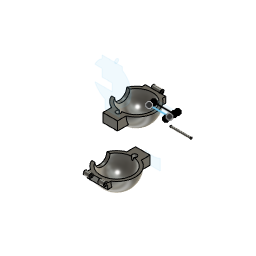
문고리 v1 (Autodesk Fusion 360 design; units mm, degrees)
Autodesk Fusion 360 part; units mm, degrees
sphere "구 기본체1" add diameter 65 placed x (1, 0, 0) y (0, 1, 0) z (0, 0, 1) at (0, 0, 0) makes body 1
split "분할1" by plane through (0, 0, 0) normal (0, 1, 0) bodies 1 makes body 2 at (30.8124, 7.6824, -6.9156)
move_body "이동1" bodies 2 to x (1, 0, 0) y (0, 1, 0) z (0, 0, 1) at (0, 40, 0)
move_body "이동2" bodies 2 to x (1, 0, 0) y (0, 1, 0) z (0, 0, 1) at (0, 80, 0)
sketch "스케치2" plane through (0, 120, 0) normal (0, -1, 0) x (1, 0, 0)
move_body "이동3" bodies 1 to x (1, 0, 0) y (0, 1, 0) z (0, 0, 1) at (190, 0, 0)
sketch "스케치3" plane through (0, 120, 0) normal (0, -1, 0) x (1, 0, 0)
  arc A0 (27.5, 0) -> (-27.5, 0) centre (0, 0) ccw
  line L0 (-27.5, 0) -> (27.5, 0)
  dimension "d2" = 27.5
  constraint coincident A0.centre origin
  constraint horizontal L0
  measures "d2" radius of A0
revolve "회전1" cut sketch "스케치3" angle 360 about axis through (-27.5, 120, 0) along (1, 0, 0) bodies 2
delete_body "본체 제거1" bodies 1
copy_body "CopyPasteBodies1" bodies 2 makes body 3
move_body "이동4" bodies 3 to x (1, 0, 0) y (0, 1, 0) z (0, 0, 1) at (130, 0, 0)
delete_body "본체 제거2" bodies 2
delete_body "본체 제거3" bodies 3
sphere "구 기본체2" add diameter 65 placed x (1, 0, 0) y (0, 1, 0) z (0, 0, 1) at (0, 0, 0) separate body makes body 4
sketch "스케치5" plane through (0, 0, 0) normal (0, 0, 1) x (1, 0, 0)
sketch "스케치6" plane through (0, 0, 0) normal (0, 0, 1) x (1, 0, 0)
  line L0 (-12.5, 0) -> (-12.5, 15)
  line L1 (-12.5, 15) -> (-12.5, -15)
  line L2 (-12.5, -15) -> (12.5, -15)
  line L3 (12.5, -15) -> (12.5, 15)
  line L4 (12.5, 15) -> (-12.5, 15)
  dimension "d7" = 12.5
  dimension "d9" = 15
  dimension "d10" = 30
  dimension "d11" = 25
  constraint perpendicular L1 L2
  constraint perpendicular L0 L4
  measures "d7" distance of origin L0.start
  measures "d9" distance of L0.start L0.end
  measures "d10" distance of L0.end L1.end
  measures "d11" distance of L1.end L2.end
extrude "돌출1" add sketch "스케치6" against normal blind 40 bodies 4
sketch "스케치7" plane through (0, 0, 0) normal (1, 0, 0) x (0, 1, 0)
  circle A0 centre (0, 0) radius 13
  dimension "d14" = 26
  constraint coincident A0.centre origin
  measures "d14" diameter of A0
extrude "돌출2" cut sketch "스케치7" against normal blind 32.5 bodies 4
extrude "돌출3" add 1 faces at (-4.1667, -5, -40) along direction (0, 0, -1) blind 10 on bodies 4 bodies 4
extrude "돌출4" cut 1 faces at (-4.1667, -5, -50) along direction (0, 0, 1) blind 5 on bodies 4 bodies 4
sketch "스케치8" plane through (0, -15, 0) normal (0, -1, 0) x (1, 0, 0)
  line L0 (-12.5, -45) -> (12.5, -45)
  line L1 (12.5, -45) -> (12.5, -25.9808)
  arc A0 (-12.5, -25.9808) -> (12.5, -25.9808) centre (0, 0) ccw
  line L2 (-12.5, -25.9808) -> (-12.5, -45)
sketch "스케치9" plane through (0, -15, 0) normal (0, -1, 0) x (1, 0, 0)
  circle A0 centre (0, -31) radius 4
  dimension "d21" = 8
  measures "d21" diameter of A0
extrude "돌출5" cut sketch "스케치9" along normal blind -65 and the other way blind -110 bodies 4
sketch "스케치10" plane through (0, 0, 0) normal (0, 0, 1) x (1, 0, 0)
  line L0 (17.5, 10) -> (-17.5, 10)
  line L1 (-17.5, 10) -> (-17.5, -10)
  line L2 (-17.5, -10) -> (17.5, -10)
  line L3 (17.5, -10) -> (17.5, 10)
  line L4 (17.5, 10) -> (-17.5, -10) construction
  line L5 (-17.5, 10) -> (17.5, -10) construction
  dimension "d26" = 35
  dimension "d27" = 20
  constraint horizontal L0
  constraint perpendicular L0 L1
  constraint parallel L0 L2
  constraint parallel L1 L3
  constraint coincident L4 origin
  constraint coincident L5 origin
  measures "d26" distance of L1.end L2.end
  measures "d27" distance of L0.end L1.end
extrude "돌출6" add sketch "스케치10" along normal blind 33 bodies 4
sketch "스케치11" plane through (0, 0, 33) normal (0, 0, 1) x (-1, 0, 0)
  line L0 (-17.5, 10) -> (-17.5, -10)
  line L1 (-17.5, -10) -> (17.5, -10)
  line L2 (17.5, -10) -> (17.5, 10)
  line L3 (17.5, 10) -> (-17.5, 10)
  line L4 (-17.5, 10) -> (-17.5, 4)
  line L5 (17.5, 4) -> (-17.5, 4)
  line L6 (-17.5, -10) -> (-17.5, -4)
  line L7 (-17.5, -4) -> (17.5, -4)
  dimension "d30" = 6
  constraint coincident L0.start L3.end
  constraint coincident L0 L4.end
  constraint perpendicular L3 L4
  constraint coincident L2 L5.start
  constraint perpendicular L4 L5
  constraint coincident L0.end L1.start
  constraint coincident L0 L6.end
  constraint coincident L2 L7.end
  constraint perpendicular L2 L7
  measures "d30" distance of L0.end L6.end
sketch "스케치12" plane through (17.5, 0, 0) normal (1, 0, 0) x (0, 1, 0)
  arc A0 (10, 25.4951) -> (-10, 25.4951) centre (0, 0) ccw
  line L0 (10, 25.4951) -> (10, 33)
  line L1 (10, 33) -> (-10, 33)
  line L2 (-10, 33) -> (-10, 25.4951)
  circle A1 centre (0, 36.5) radius 3.5
split "분할2" by plane through (0, 0, 0) normal (0, 1, 0) bodies 4 makes body 5 at (28.1333, 16.2428, -0.9692)
move_body "이동5" bodies 5 to x (1, 0, 0) y (0, 1, 0) z (0, 0, 1) at (-115, 30, 0)
sketch "스케치13" plane through (0, 30, 0) normal (0, -1, 0) x (1, 0, 0)
  line L0 (-127.5, -45) -> (-102.5, -45)
  line L1 (-102.5, -45) -> (-102.5, -30)
  arc A0 (-102.5, -30) -> (-97.5, 27.3861) centre (-115, 0) ccw
  line L2 (-97.5, 27.3861) -> (-97.5, 33)
  line L3 (-97.5, 33) -> (-132.5, 33)
  line L4 (-132.5, 33) -> (-132.5, 27.3861)
  arc A1 (-132.5, 27.3861) -> (-144.7867, 13) centre (-115, 0) ccw
  line L5 (-144.7867, 13) -> (-132.5, 13)
  line L6 (-132.5, 13) -> (-132.5, 0)
  line L7 (-132.5, 0) -> (-115, 0)
  line L8 (-115, 0) -> (-115, -13)
  line L9 (-115, -13) -> (-144.7867, -13)
  arc A2 (-144.7867, -13) -> (-127.5, -30) centre (-115, 0) ccw
  line L10 (-127.5, -30) -> (-127.5, -45)
  circle A3 centre (-115, -31) radius 4
sketch "스케치14" plane through (0, 30, 0) normal (0, -1, 0) x (1, 0, 0)
  arc A0 (-87.5, 0) -> (-142.5, 0) centre (-115, 0) ccw
  line L0 (-142.5, 0) -> (-87.5, 0)
  dimension "d31" = 27.5
  constraint horizontal L0
  measures "d31" radius of A0
sketch "스케치15" plane through (0, 30, 0) normal (0, -1, 0) x (1, 0, 0)
sketch "스케치16" plane through (0, 30, 0) normal (0, -1, 0) x (1, 0, 0)
revolve "회전2" cut sketch "스케치14" angle 360 about axis through (-142.5, 30, 0) along (1, 0, 0) bodies 5
sketch "스케치17" plane through (0, 0, 0) normal (0, 1, 0) x (-1, 0, 0)
  circle A0 centre (0, -31) radius 4
  line L0 (-12.5, -45) -> (12.5, -45)
  line L1 (12.5, -45) -> (12.5, -30)
  arc A1 (12.5, -30) -> (29.7867, -13) centre (0, 0) ccw
  line L2 (29.7867, -13) -> (0, -13)
  line L3 (0, -13) -> (0, 0)
  line L4 (0, 0) -> (17.5, 0)
  line L5 (17.5, 0) -> (17.5, 13)
  line L6 (17.5, 13) -> (29.7867, 13)
  arc A2 (29.7867, 13) -> (17.5, 27.3861) centre (0, 0) ccw
  line L7 (17.5, 27.3861) -> (17.5, 33)
  line L8 (17.5, 33) -> (-17.5, 33)
  line L9 (-17.5, 33) -> (-17.5, 27.3861)
  arc A3 (-17.5, 27.3861) -> (-12.5, -30) centre (0, 0) ccw
  line L10 (-12.5, -30) -> (-12.5, -45)
  arc A4 (27.5, 0) -> (-27.5, 0) centre (0, 0) ccw
  line L11 (-27.5, 0) -> (27.5, 0)
  dimension "d33" = 27.5
  constraint coincident A1.centre L3.end
  constraint parallel L2 L11
  measures "d33" radius of A4
revolve "회전3" cut sketch "스케치17" angle 360 about axis through (27.5, 0, 0) along (-1, 0, 0) contours L4 L5 L6 A4 L11 bodies 4
sketch "스케치18" plane through (17.5, 0, 0) normal (1, 0, 0) x (0, 1, 0)
sketch "스케치19" plane through (-97.5, 0, 0) normal (1, 0, 0) x (0, 1, 0)
  line L0 (30, 33) -> (30, 27.3861)
  arc A0 (40, 25.4951) -> (30, 27.3861) centre (30, 0) ccw
  line L1 (40, 25.4951) -> (40, 33)
  line L2 (40, 33) -> (30, 33)
  circle A1 centre (30, 36.5) radius 3.5
  dimension "d35" = 7
  constraint coincident L0.start A1
  measures "d35" diameter of A1
extrude "돌출7" add sketch "스케치12" against normal blind 9.8 separate body contours A1 makes body 6
sketch "스케치20" plane through (-17.5, 0, 0) normal (-1, 0, 0) x (0, -1, 0)
  line L0 (0, 33) -> (0, 27.3861)
  arc A0 (10, 25.4951) -> (0, 27.3861) centre (0, 0) ccw
  line L1 (10, 25.4951) -> (10, 33)
  line L2 (10, 33) -> (0, 33)
  circle A1 centre (0, 36.5) radius 3.5
  constraint coincident L0.start A1
extrude "돌출8" add sketch "스케치20" against normal blind 9.8 separate body contours A1 makes body 7
sketch "스케치21" plane through (0, 0, 33) normal (0, 0, 1) x (-1, 0, 0)
sketch "스케치22" plane through (0, 0, 33) normal (0, 0, 1) x (-1, 0, 0)
sketch "스케치23" plane through (0, 0, 33) normal (0, 0, 1) x (-1, 0, 0)
sketch "스케치24" plane through (0, 0, 33) normal (0, 0, 1) x (-1, 0, 0)
  line L0 (-17.5, 0) -> (-7.7, 0)
  line L1 (-7.7, 0) -> (-7.7, 3.4545)
  line L2 (-7.7, 3.4545) -> (-17.5, 3.4545)
  line L3 (-17.5, 3.4545) -> (-17.5, 0)
  dimension "d40" = 9.8
  constraint horizontal L0
  constraint vertical L1
  constraint horizontal L2
  constraint vertical L3
  measures "d40" distance of L0.start L0.end
extrude "돌출9" add sketch "스케치24" along normal blind 3 bodies 6 7 4
sketch "스케치25" plane through (0, 0, 33) normal (0, 0, 1) x (-1, 0, 0)
  line L0 (17.5, 0) -> (7.7, 0)
  line L1 (7.7, 0) -> (7.7, 3.4802)
  line L2 (7.7, 3.4802) -> (17.5, 3.4802)
  line L3 (17.5, 3.4802) -> (17.5, 0)
  dimension "d43" = 9.8
  constraint horizontal L0
  constraint vertical L1
  constraint horizontal L2
  constraint vertical L3
  measures "d43" distance of L0.start L0.end
extrude "돌출10" add sketch "스케치25" along normal blind 4 bodies 7 6
extrude "돌출11" add sketch "스케치19" against normal blind 35 separate body contours A1 makes body 8
extrude "돌출12" cut 1 faces at (-97.5, 29.7193, 37.5761) along direction (-1, 0, 0) blind 10 on bodies 8 bodies 8
extrude "돌출13" cut 1 faces at (-132.5, 28.7534, 35.5879) along direction (1, 0, 0) blind 10 on bodies 8 bodies 8
sketch "스케치26" plane through (0, 0, 33) normal (0, 0, 1) x (-1, 0, 0)
  line L0 (132.5, -30) -> (97.5, -30)
  line L1 (97.5, -30) -> (97.5, -40)
  line L2 (97.5, -40) -> (132.5, -40)
  line L3 (132.5, -40) -> (132.5, -30)
  line L4 (122.5015, -30) -> (107.5469, -30)
  line L5 (107.5469, -30) -> (107.5469, -33.3747)
  line L6 (107.5469, -33.3747) -> (122.5015, -33.3747)
  line L7 (122.5015, -33.3747) -> (122.5015, -30)
  constraint horizontal L4
  constraint vertical L5
  constraint horizontal L6
  constraint vertical L7
  constraint coincident L0 L4.start
extrude "돌출14" add sketch "스케치26" along normal blind 4.5 contours L0 L4 L5 L6 L7 bodies 8 5
sketch "스케치27" plane through (0, 0, 33) normal (0, 0, 1) x (-1, 0, 0)
sketch "스케치28" plane through (17.5, 0, 0) normal (1, 0, 0) x (0, 1, 0)
  line L0 (0, 27.3861) -> (0, 33)
  arc A0 (0, 33) -> (-3.4545, 35.9373) centre (0, 36.5) ccw
  line L1 (-3.4545, 35.9373) -> (-3.4545, 33)
  line L2 (-3.4545, 33) -> (-10, 33)
  line L3 (-10, 33) -> (-10, 25.4951)
  arc A1 (0, 27.3861) -> (-10, 25.4951) centre (0, 0) ccw
  circle A2 centre (0, 36.5) radius 1.75
  dimension "d54" = 3.5
  constraint concentric A0 A2
  measures "d54" diameter of A2
extrude "돌출15" cut sketch "스케치28" against normal blind 43 contours A2 bodies 7
sketch "스케치29" plane through (-107.5, 0, 0) normal (1, 0, 0) x (0, 1, 0)
  circle A0 centre (30, 36.5) radius 3.5
sketch "스케치30" plane through (-107.5, 0, 0) normal (1, 0, 0) x (0, 1, 0)
  circle A0 centre (30, 36.5) radius 1.75
  dimension "d57" = 3.5
  measures "d57" diameter of A0
extrude "돌출16" cut sketch "스케치30" against normal blind 50 bodies 8
sketch "스케치31" plane through (0, 0, 0) normal (0, 0, 1) x (1, 0, 0)
sketch "스케치32" plane through (0, 0, 0) normal (1, 0, 0) x (0, 1, 0)
  circle A0 centre (15.6993, 0) radius 1.7
  dimension "d60" = 3.4
  measures "d60" diameter of A0
extrude "돌출17" add sketch "스케치32" along normal blind 35 separate body makes body 9
move_body "이동6" bodies 8 to x (1, 0, 0) y (0, 0, -1) z (0, 1, 0) at (0, 71.5, -18.5)
move_body "이동7" bodies 7 to x (1, 0, 0) y (0, 0, 1) z (0, -1, 0) at (0, -77.5, -12.5)
